Autodesk Fusion 360 part; units mm, degrees
note: some values were not read from the file. Chosen so that the rebuilt part matches the saved one: which bodies a step acts on.
(part 2 of 2)
sketch "TOP (2)" plane through (0, 0, 120) normal (0, 0, 1) x (-1, 0, 0)
  line L0 (-129.8845, -80.1297) -> (-129.8845, -19.9324)
  line L1 (-129.8845, -19.9324) -> (-19.9408, -19.9324)
  line L2 (-19.9408, -19.9324) -> (-19.9408, -80.1297)
  line L3 (-19.9408, -80.1297) -> (-129.8845, -80.1297)
  line L4 (-180.5, -80.1297) -> (-180.5, -19.5144)
  line L5 (-180.5, -19.5144) -> (-169.4021, -19.5144)
  line L6 (-159.565, -19.5144) -> (-159.565, -80.1297)
  line L7 (-159.565, -80.1297) -> (-180.5, -80.1297)
  line L8 (-151.5, -18.5714) -> (-148.5, -18.5714)
  line L9 (-148.5, -18.5714) -> (-148.5, -37.1429)
  line L10 (-148.5, -37.1429) -> (-151.5, -37.1429)
  line L11 (-151.5, -37.1429) -> (-151.5, -18.5714)
  line L12 (-151.5, -55.7143) -> (-148.5, -55.7143)
  line L13 (-148.5, -55.7143) -> (-148.5, -74.2857)
  line L14 (-148.5, -74.2857) -> (-151.5, -74.2857)
  line L15 (-151.5, -74.2857) -> (-151.5, -55.7143)
  line L16 (-300, -55.7143) -> (-297, -55.7143)
  line L17 (-297, -55.7143) -> (-297, -74.2857)
  line L18 (-297, -74.2857) -> (-300, -74.2857)
  line L19 (-300, -111.4286) -> (-300, -130)
  line L20 (-300, -130) -> (-280, -130)
  line L21 (-280, -130) -> (-280, -127)
  line L22 (-280, -127) -> (-260, -127)
  line L23 (-260, -127) -> (-260, -130)
  line L24 (-260, -130) -> (-240, -130)
  line L25 (-240, -130) -> (-240, -127)
  line L26 (-240, -127) -> (-220, -127)
  line L27 (-220, -127) -> (-220, -130)
  line L28 (-220, -130) -> (-200, -130)
  line L29 (-200, -130) -> (-200, -127)
  line L30 (-200, -127) -> (-180, -127)
  line L31 (-180, -127) -> (-180, -130)
  line L32 (-180, -130) -> (-160, -130)
  line L33 (-160, -130) -> (-160, -127)
  line L34 (-160, -127) -> (-140, -127)
  line L35 (-140, -127) -> (-140, -130)
  line L36 (-140, -130) -> (-120, -130)
  line L37 (-120, -130) -> (-120, -127)
  line L38 (-120, -127) -> (-100, -127)
  line L39 (-100, -127) -> (-100, -130)
  line L40 (-100, -130) -> (-80, -130)
  line L41 (-80, -130) -> (-80, -127)
  line L42 (-80, -127) -> (-60, -127)
  line L43 (-60, -127) -> (-60, -130)
  line L44 (-60, -130) -> (-40, -130)
  line L45 (-40, -130) -> (-40, -127)
  line L46 (-40, -127) -> (-20, -127)
  line L47 (-20, -127) -> (-20, -130)
  line L48 (-20, -130) -> (0, -130)
  line L49 (0, -130) -> (0, -111.4286)
  line L50 (0, -74.2857) -> (-3, -74.2857)
  line L51 (-3, -74.2857) -> (-3, -55.7143)
  line L52 (-3, -55.7143) -> (0, -55.7143)
  line L53 (0, -55.7143) -> (0, -37.1429)
  line L54 (0, -37.1429) -> (-3, -37.1429)
  line L55 (-3, -37.1429) -> (-3, -18.5714)
  line L56 (-3, -18.5714) -> (0, -18.5714)
  line L57 (0, -18.5714) -> (0, 0)
  line L58 (0, 0) -> (-20, 0)
  line L59 (-20, 0) -> (-20, -3)
  line L60 (-20, -3) -> (-40, -3)
  line L61 (-40, -3) -> (-40, 0)
  line L62 (-40, 0) -> (-60, 0)
  line L63 (-60, 0) -> (-60, -3)
  line L64 (-60, -3) -> (-80, -3)
  line L65 (-80, -3) -> (-80, 0)
  line L66 (-80, 0) -> (-100, 0)
  line L67 (-100, 0) -> (-100, -3)
  line L68 (-100, -3) -> (-120, -3)
  line L69 (-120, -3) -> (-120, 0)
  line L70 (-120, 0) -> (-140, 0)
  line L71 (-140, 0) -> (-140, -3)
  line L72 (-140, -3) -> (-160, -3)
  line L73 (-160, -3) -> (-160, 0)
  line L74 (-160, 0) -> (-180, 0)
  line L75 (-180, 0) -> (-180, -3)
  line L76 (-180, -3) -> (-200, -3)
  line L77 (-200, -3) -> (-200, 0)
  line L78 (-200, 0) -> (-220, 0)
  line L79 (-220, 0) -> (-220, -3)
  line L80 (-220, -3) -> (-240, -3)
  line L81 (-240, -3) -> (-240, 0)
  line L82 (-240, 0) -> (-260, 0)
  line L83 (-260, 0) -> (-260, -3)
  line L84 (-260, -3) -> (-280, -3)
  line L85 (-280, -3) -> (-280, 0)
  line L86 (-280, 0) -> (-300, 0)
  line L87 (-300, 0) -> (-300, -18.5714)
  line L88 (-300, -18.5714) -> (-297, -18.5714)
  line L89 (-297, -18.5714) -> (-297, -37.1429)
  line L90 (-297, -37.1429) -> (-300, -37.1429)
  line L91 (-300, -37.1429) -> (-300, -55.7143)
  line L92 (-169.4021, -19.5144) -> (-169.4021, -19.1021)
  line L93 (-169.4021, -19.1021) -> (-161.4021, -19.1021)
  line L94 (-161.4021, -19.1021) -> (-161.4021, -19.5144)
  line L95 (-161.4021, -19.5144) -> (-159.565, -19.5144)
  line L96 (-284.4296, -73.3855) -> (-284.4296, -19.3855)
  line L97 (-284.4296, -19.3855) -> (-183.4296, -19.3855)
  line L98 (-183.4296, -19.3855) -> (-183.4296, -73.3855)
  line L99 (-183.4296, -73.3855) -> (-284.4296, -73.3855)
  line L100 (-270.7569, -113.0322) -> (-270.7569, -90.0322)
  line L101 (-270.7569, -90.0322) -> (-199.7569, -90.0322)
  line L102 (-199.7569, -90.0322) -> (-199.7569, -113.0322)
  line L103 (-199.7569, -113.0322) -> (-270.7569, -113.0322)
  circle A0 centre (-125.8569, -100.5311) radius 5
  line L104 (-151.5, -92.8571) -> (-148.5, -92.8571)
  line L105 (-148.5, -92.8571) -> (-148.5, -111.4286)
  line L106 (-148.5, -111.4286) -> (-151.5, -111.4286)
  line L107 (-151.5, -111.4286) -> (-151.5, -92.8571)
  line L108 (-300, -92.8571) -> (-297, -92.8571)
  line L109 (-297, -92.8571) -> (-297, -111.4286)
  line L110 (-297, -111.4286) -> (-300, -111.4286)
  line L111 (0, -111.4286) -> (-3, -111.4286)
  line L112 (-3, -111.4286) -> (-3, -92.8571)
  line L113 (-3, -92.8571) -> (0, -92.8571)
  line L114 (0, -92.8571) -> (0, -74.2857)
  line L115 (-300, -74.2857) -> (-300, -92.8571)
sketch "BOTTOM (2)" plane through (0, 0, 0) normal (0, 0, -1) x (1, 0, 0)
  line L0 (297, -55.7143) -> (300, -55.7143)
  line L1 (300, -55.7143) -> (300, -37.1429)
  line L2 (300, -37.1429) -> (297, -37.1429)
  line L3 (297, -37.1429) -> (297, -18.5714)
  line L4 (297, -18.5714) -> (300, -18.5714)
  line L5 (300, -18.5714) -> (300, 0)
  line L6 (300, 0) -> (280, 0)
  line L7 (280, 0) -> (280, -3)
  line L8 (280, -3) -> (260, -3)
  line L9 (260, -3) -> (260, 0)
  line L10 (260, 0) -> (240, 0)
  line L11 (240, 0) -> (240, -3)
  line L12 (240, -3) -> (220, -3)
  line L13 (220, -3) -> (220, 0)
  line L14 (220, 0) -> (200, 0)
  line L15 (200, 0) -> (200, -3)
  line L16 (200, -3) -> (180, -3)
  line L17 (180, -3) -> (180, 0)
  line L18 (180, 0) -> (160, 0)
  line L19 (160, 0) -> (160, -3)
  line L20 (160, -3) -> (140, -3)
  line L21 (140, -3) -> (140, 0)
  line L22 (140, 0) -> (120, 0)
  line L23 (120, 0) -> (120, -3)
  line L24 (120, -3) -> (100, -3)
  line L25 (100, -3) -> (100, 0)
  line L26 (100, 0) -> (80, 0)
  line L27 (80, 0) -> (80, -3)
  line L28 (80, -3) -> (60, -3)
  line L29 (60, -3) -> (60, 0)
  line L30 (60, 0) -> (40, 0)
  line L31 (40, 0) -> (40, -3)
  line L32 (40, -3) -> (20, -3)
  line L33 (20, -3) -> (20, 0)
  line L34 (20, 0) -> (0, 0)
  line L35 (0, 0) -> (0, -18.5714)
  line L36 (0, -18.5714) -> (3, -18.5714)
  line L37 (3, -18.5714) -> (3, -37.1429)
  line L38 (3, -37.1429) -> (0, -37.1429)
  line L39 (0, -37.1429) -> (0, -55.7143)
  line L40 (0, -55.7143) -> (3, -55.7143)
  line L41 (3, -55.7143) -> (3, -74.2857)
  line L42 (3, -74.2857) -> (0, -74.2857)
  line L43 (0, -111.4286) -> (0, -130)
  line L44 (0, -130) -> (20, -130)
  line L45 (20, -130) -> (20, -127)
  line L46 (20, -127) -> (40, -127)
  line L47 (40, -127) -> (40, -130)
  line L48 (40, -130) -> (60, -130)
  line L49 (60, -130) -> (60, -127)
  line L50 (60, -127) -> (80, -127)
  line L51 (80, -127) -> (80, -130)
  line L52 (80, -130) -> (100, -130)
  line L53 (100, -130) -> (100, -127)
  line L54 (100, -127) -> (120, -127)
  line L55 (120, -127) -> (120, -130)
  line L56 (120, -130) -> (140, -130)
  line L57 (140, -130) -> (140, -127)
  line L58 (140, -127) -> (160, -127)
  line L59 (160, -127) -> (160, -130)
  line L60 (160, -130) -> (180, -130)
  line L61 (180, -130) -> (180, -127)
  line L62 (180, -127) -> (200, -127)
  line L63 (200, -127) -> (200, -130)
  line L64 (200, -130) -> (220, -130)
  line L65 (220, -130) -> (220, -127)
  line L66 (220, -127) -> (240, -127)
  line L67 (240, -127) -> (240, -130)
  line L68 (240, -130) -> (260, -130)
  line L69 (260, -130) -> (260, -127)
  line L70 (260, -127) -> (280, -127)
  line L71 (280, -127) -> (280, -130)
  line L72 (280, -130) -> (300, -130)
  line L73 (300, -92.8571) -> (300, -74.2857)
  line L74 (300, -74.2857) -> (297, -74.2857)
  line L75 (297, -74.2857) -> (297, -55.7143)
  line L76 (148.5, -55.7143) -> (151.5, -55.7143)
  line L77 (151.5, -55.7143) -> (151.5, -74.2857)
  line L78 (151.5, -74.2857) -> (148.5, -74.2857)
  line L79 (148.5, -74.2857) -> (148.5, -55.7143)
  line L80 (148.5, -18.5714) -> (151.5, -18.5714)
  line L81 (151.5, -18.5714) -> (151.5, -37.1429)
  line L82 (151.5, -37.1429) -> (148.5, -37.1429)
  line L83 (148.5, -37.1429) -> (148.5, -18.5714)
  line L84 (297, -92.8571) -> (300, -92.8571)
  line L85 (0, -74.2857) -> (0, -92.8571)
  line L86 (0, -92.8571) -> (3, -92.8571)
  line L87 (3, -92.8571) -> (3, -111.4286)
  line L88 (3, -111.4286) -> (0, -111.4286)
  line L89 (300, -130) -> (300, -111.4286)
  line L90 (300, -111.4286) -> (297, -111.4286)
  line L91 (297, -111.4286) -> (297, -92.8571)
  line L92 (148.5, -92.8571) -> (151.5, -92.8571)
  line L93 (151.5, -92.8571) -> (151.5, -111.4286)
  line L94 (151.5, -111.4286) -> (148.5, -111.4286)
  line L95 (148.5, -111.4286) -> (148.5, -92.8571)
component "Main Box" placed x (1, 0, 0) y (0, 1, 0) z (0, 0, 1) at (0, 0, 0)
component "Dividers" placed x (1, 0, 0) y (0, 1, 0) z (0, 0, 1) at (0, 0, 0)
hidden bodies 7
equation "length = 300 mm" comment "User defined length of the box"
equation "width = 130 mm" comment "User defined width of the box"
equation "height = 120 mm" comment "User defined height of the box"
equation "thickness = 3 mm" comment "User defined thickness of the outer box material"
equation "ciheight = height - thickness" comment "Calculated inner height of the box"
equation "ciwidth = width - thickness * 2" comment "Calculated inner width of the box"
equation "cilength = length - thickness * 2" comment "Calculated inner length of the box"
equation "fingerw = thickness * 6" comment "Optimal finger width"
equation "lfingers = max(3; ( floor(ceil(length / fingerw) / 2) * 2 ) - 1)" comment "Length axis: number of fingers"
equation "lfingerw = length / lfingers" comment "Length axis: actual finger width"
equation "lnotches = floor(lfingers / 2)" comment "Length axis: number of notches along the edge"
equation "lnotchl = ( lfingers - 2 ) * lfingerw" comment "Length axis: length of the notch reference line"
equation "wfingers = max(3; ( floor(ceil(width / fingerw) / 2) * 2 ) - 1)" comment "Width axis: number of fingers"
equation "wfingerw = width / wfingers" comment "Width axis: actual finger width"
equation "wnotches = floor(wfingers / 2)" comment "Width axis: number of notches along the edge"
equation "wnotchl = ( wfingers - 2 ) * wfingerw" comment "Width axis: length of the notch reference line"
equation "hfingers = max(3; ( floor(ceil(ciheight / fingerw) / 2) * 2 ) - 1)" comment "Height axis: number of fingers"
equation "hfingerw = ciheight / hfingers" comment "Height axis: actual finger width"
equation "hnotches = floor(hfingers / 2)" comment "Height axis: number of notches along the edge"
equation "hnotchl = ( hfingers - 2 ) * hfingerw" comment "Height axis: length of the notch reference line"
equation "d21 = length"
equation "d22 = width"
equation "d23 = thickness"
equation "d25 = lfingerw"
equation "d26 = lnotchl"
equation "d27 = -thickness"
equation "d29 = lnotches"
equation "d31 = lnotchl - lfingerw"
equation "d32 = width - thickness"
equation "d33 = wfingerw"
equation "d34 = wnotchl"
equation "d35 = -thickness"
equation "d37 = wnotches"
equation "d38 = 2 + cldividers"
equation "d39 = wnotchl - wfingerw"
equation "d40 = -( length - thickness )"
equation "d41 = length"
equation "d42 = height"
equation "d43 = thickness"
equation "d45 = thickness"
equation "d46 = hfingerw"
equation "d47 = hnotchl"
equation "d48 = -thickness"
equation "d50 = hnotches"
equation "d51 = 2 + cldividers"
equation "d52 = hnotchl - hfingerw"
equation "d53 = length - thickness"
equation "d56 = width - thickness"
equation "d58 = width"
equation "d59 = height"
equation "d60 = thickness"
equation "d62 = 2 + cldividers"
equation "d64 = length - thickness"
equation "lcompartments = ldividers + 1" comment "Length axis: Number of compartments"
equation "clcompartments = max(0; lcompartments)" comment "Length axis: Calculated number of compartments"
equation "cldividers = max(0; clcompartments - 1)" comment "Length axis: Number of dividers"
equation "wcompartments = wdividers + 1" comment "Width axis: number of compartments"
equation "cwcompartments = max(0; wcompartments)" comment "Width axis: calculated number of compartments"
equation "cwdividers = max(0; cwcompartments - 1)" comment "Width axis: calculated number of dividers"
equation "d72 = hfingerw"
equation "d73 = -thickness"
equation "d75 = 2 + cwdividers"
equation "d77 = width - thickness"
equation "cwspacing = ( width - thickness ) / cwcompartments" comment "Width axis: Spacing between dividers"
equation "ldividers = 1" comment "Length axis: number of dividers"
equation "wdividers = 0" comment "Width axis: number of dividers"
equation "dividero = 50 mm" comment "Divider offset from main box"
equation "d98 = height - thickness"
equation "d100 = height - thickness - thickness"
equation "d101 = thickness"
equation "d103 = -thickness"
equation "d107 = -thickness"
equation "d115 = -thickness"
equation "d117 = -thickness"
named bodies: "Bottom Panel", "Front Panel", "Back Panel", "Left Panel", "Left Panel (1)", "Left Panel (2)"
